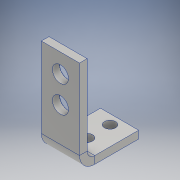
# Autodesk Inventor part: Część4
Saved by Autodesk Inventor 2019.4 (Build 234330000, 330)
## iProperties
Created: 2019-05-25
Part Number: Część4
Material: Aluminium 6061
Document SubType Name: Konstrukcja blachowa
Designer: barto
Density: 2.7 g/cm^3
Flat Pattern Width: 1 cm
Flat Pattern Length: 3.70239 cm
Flat Pattern Area: 3.70239 cm^2
Sheet Metal Rule: Domyślny_mm
Sheet Metal Width: 10,000 mm
Sheet Metal Length: 37,024 mm
Sheet Metal Area: 370,239 mm^2
Appearance: Aluminium — płaski
Author: barto
Autodesk Inventor part; units mm, degrees
ref_plane "YZ Plane" through (0, 0, 0) normal (1, 0, 0) x (0, 1, 0)
ref_plane "XZ Plane" through (0, 0, 0) normal (0, 1, 0) x (-1, 0, 0)
ref_plane "XY Plane" through (0, 0, 0) normal (0, 0, 1) x (1, 0, 0)
sketch "Szkic1" plane through (0, 0, 0) normal (0, 1, 0) x (-1, 0, 0)
  line L0 (10, 0) -> (0, 0)
  line L1 (0, 0) -> (0, -25)
  line L2 (0, -25) -> (10, -25)
  line L3 (10, -25) -> (10, 0)
  dimension "d0" = 25
  dimension "d1" = 10
  dimension "d13" = 0
  dimension "d14" = 0
  measures "d0" distance of L2.end L0.start
  measures "d1" distance of L1.end L2.end
  measures "d13" distance from line of point (0, 0) L0
  measures "d14" distance from line of L1 point (0, 0)
extrude "Płyta1" add sketch "Szkic1" along normal blind 2
sketch "Szkic2" plane through (-10, 0, -23) normal (0, 0, -1) x (-1, 0, 0)
  line L0 (-10, 0) -> (0, 0)
  line L1 (0, 0) -> (0, 15.5)
  line L2 (0, 15.5) -> (-10, 15.5)
  line L3 (-10, 15.5) -> (-10, 0)
  constraints: 6 end point, 1 horizontal, 1 perpendicular, 1 vertical
edge flange "Kołnierz1" height 15.5 angle 90 thickness 2 bend radius 2 thickness toward (0, 0, -1) relief tear relief width 2 relief depth 1 edges at (-5, 2, -25) wall of the first edge with corners at (0, 0, -23) (-10, 0, -23) (-10, 15.5, -23) (0, 15.5, -23)
bend "Zagięcie1"
corner "Narożnik1"
sketch "Szkic4" plane through (0, 2, 0) normal (0, 1, 0) x (1, 0, 0)
  line L0 (-10, 0) -> (-10, 21) projected
  line L1 (0, 0) -> (-10, 0) projected
  point P0 (-5, 5)
  point P1 (-5, 12)
  dimension "d48" = 5
  dimension "d49" = 7
  measures "d48" distance from line of L1 point (-5, 5)
  measures "d49" distance of point (-5, 12) point (-5, 5)
sketch "Szkic5" plane through (-10, 15.5, -23) normal (0, 0, 1) x (1, 0, 0)
  line L0 (10, 0) -> (0, 0) projected
  line L1 (0, 0) -> (0, -11.5) projected
  point P0 (10, -15.5)
  point P1 (5, -8.5)
  point P2 (5, -2.5)
  dimension "d50" = 6
  dimension "d51" = 2.5
  measures "d50" distance of point (5, -8.5) point (5, -2.5)
  measures "d51" distance from line of L0 point (5, -2.5)
hole "Otwór1" at (-5, 7, -23) at (-5, 13, -23) direction (0, 0, -1) diameter 2.9 end through all clearance for "Wkręt z łbem walcowym gniazdowym ISO 4762" size "M2.5" standard "ISO"
hole "Otwór2" at (-5, 2, -5) at (-5, 2, -12) direction (0, -1, 0) diameter 4.22 end through all
chamfer "Faza1" distance 0.1 angle 45 2 edges at (-5, 2, -7.11) (-5, 2, -14.11)
equation "\"d36\" = Grubość"
equation "\"d43\" = Grubość"
equation "\"d2\" = Grubość"
equation "\"d3\" = SzerokośćGięciaPodcięcia"
equation "\"d4\" = GłębokośćGięciaPodcięcia"
equation "\"d5\" = MinimalnaPozostałość"
equation "\"d6\" = PromieńPrzejścia"
equation "\"d9\" = PromieńGięcia"
equation "\"d10\" = RozmiarPodcięciaNarożnika"
equation "\"d11\" = Wielk_odstępu"
equation "\"d12\" = Rozmiar_promienia_Jacobiego"
equation "\"PromieńGięcia\" = Grubość"
equation "\"SzerokośćGięciaPodcięcia\" = Grubość"
equation "\"GłębokośćGięciaPodcięcia\" = 0.5 * Grubość"
equation "\"RozmiarPodcięciaNarożnika\" = 4 * Grubość"
equation "\"MinimalnaPozostałość\" = 2 * Grubość"
equation "\"PromieńPrzejścia\" = PromieńGięcia"
equation "\"Rozmiar_promienia_Jacobiego\" = PromieńGięcia"
equation "\"Wielk_odstępu\" = Grubość"
equation "\"Grubość\" = 2"
